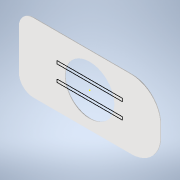
# Autodesk Inventor part: Bodenplatte-Holz
Saved by Autodesk Inventor 2020.3 (Build 243373010, 373A)
## iProperties
Created: 2021-01-31
Part Number: Bodenplatte-Holz
Material: Generisch
Document SubType Name: Modeling
Designer: Stefan
Density: 1 g/cm^3
Appearance: Vorgabe
Author: Stefan
Autodesk Inventor part; units mm, degrees
ref_plane "YZ Plane" through (0, 0, 0) normal (1, 0, 0) x (0, 1, 0)
ref_plane "XZ Plane" through (0, 0, 0) normal (0, 1, 0) x (-1, 0, 0)
ref_plane "XY Plane" through (0, 0, 0) normal (0, 0, 1) x (1, 0, 0)
sketch "Skizze2" plane through (0, 0, 0) normal (0, 0, 1) x (1, 0, 0)
  line L0 (-775, 475) -> (575, 475)
  line L1 (975, 75) -> (975, -75)
  line L2 (575, -475) -> (-775, -475)
  line L3 (-975, -275) -> (-975, 275)
  arc A0 (975, 75) -> (575, 475) centre (575, 75) ccw
  arc A1 (575, -475) -> (975, -75) centre (575, -75) ccw
  arc A2 (-775, 475) -> (-975, 275) centre (-775, 275) ccw
  arc A3 (-975, -275) -> (-775, -475) centre (-775, -275) ccw
  circle A4 centre (0, 0) radius 340
  point P0 (975, -475)
  point P1 (975, 475)
  point P2 (-975, -475)
  dimension "d0" = 950
  dimension "d1" = 1950
  dimension "d2" = 400
  dimension "d3" = 200
  dimension "d4" = 680
  dimension "d5" = 975
  dimension "d6" = 475
  constraints: 8 end point, 8 point on circle, 8 tangent, 6 point on line, 5 centre point, 2 equal radius, 2 parallel, 1 coincident, 1 horizontal, 1 perpendicular
  measures "d0" distance of point (975, 475) point (975, -475)
  measures "d1" distance of point (975, -475) point (-975, -475)
  measures "d2" radius of A0
  measures "d3" radius of A2
  measures "d4" diameter of A4
  measures "d5" distance from line of L1 A4.centre
  measures "d6" distance from line of L0 A4.centre
extrude "Extrusion1" add sketch "Skizze2" along normal blind 10
sketch "Skizze3" plane through (0, 0, 10) normal (0, 0, 1) x (1, 0, 0)
  line L0 (-450, -90) -> (450, -90)
  line L1 (450, -90) -> (450, -130)
  line L2 (450, -130) -> (-450, -130)
  line L3 (-450, -130) -> (-450, -90)
  line L4 (-450, 130) -> (450, 130)
  line L5 (450, 130) -> (450, 90)
  line L6 (450, 90) -> (-450, 90)
  line L7 (-450, 90) -> (-450, 130)
  point P0 (0, 0)
  dimension "d9" = 900
  dimension "d10" = 40
  dimension "d11" = 450
  dimension "d12" = 90
  dimension "d13" = 900
  dimension "d14" = 40
  dimension "d15" = 450
  dimension "d16" = 90
  constraints: 16 end point, 4 parallel, 2 horizontal, 2 perpendicular
  measures "d9" distance of L1.end L2.end
  measures "d10" distance of L0.end L1.end
  measures "d11" distance from line of point (0, 0) L1
  measures "d12" distance from line of point (0, 0) L0
  measures "d13" distance of L5.end L6.end
  measures "d14" distance of L4.end L5.end
  measures "d15" distance from line of point (0, 0) L5
  measures "d16" distance from line of point (0, 0) L6
